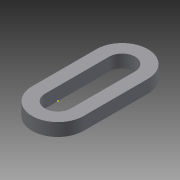
# Autodesk Inventor part: 3-2
Saved by Autodesk Inventor 2015 (Build 190159000, 159)
## iProperties
Created: 2015-09-09
Part Number: 3-2
Material: Generic
Document SubType Name: Modeling
Designer: Brandon
Density: 1 g/cm^3
Appearance: Default
Author: Brandon
Autodesk Inventor part; units mm, degrees
ref_plane "YZ Plane" through (0, 0, 0) normal (1, 0, 0) x (0, 1, 0)
ref_plane "XZ Plane" through (0, 0, 0) normal (0, 1, 0) x (-1, 0, 0)
ref_plane "XY Plane" through (0, 0, 0) normal (0, 0, 1) x (1, 0, 0)
sketch "Sketch1" plane through (0, 0, 0) normal (0, 1, 0) x (-1, 0, 0)
  circle A0 centre (0, 0) radius 25.4
  circle A1 centre (0, -63.5) radius 25.4
  line L0 (25.4, 0) -> (-25.4, 0)
  line L1 (-25.4, 0) -> (-25.4, -63.5)
  line L2 (-25.4, -63.5) -> (25.4, -63.5)
  line L3 (25.4, -63.5) -> (25.4, 0)
  dimension "d0" = 50.8
  dimension "d1" = 50.8
  dimension "d2" = 63.5
  constraints: 8 end point, 2 horizontal alignment, 2 parallel, 1 coincident, 1 horizontal, 1 perpendicular, 4 other
  measures "d2" distance of point (0, -63.5) point (0, 0)
extrude "Extrusion1" add sketch "Sketch1" along normal blind 12.7
sketch "Sketch2" plane through (0, 12.7, 0) normal (0, 1, 0) x (1, 0, 0)
  point P0 (0, 0)
sketch "Sketch3" plane through (0, 12.7, 0) normal (0, 1, 0) x (1, 0, 0)
  point P0 (0, 0)
sketch "Sketch4" plane through (0, 12.7, 0) normal (0, 1, 0) x (1, 0, 0)
  circle A0 centre (0, 0) radius 12.7
  arc A1 (-25.4, 0) -> (25.4, 0) centre (0, 0) ccw projected
  line L0 (0, 0) -> (0, 63.5)
  circle A2 centre (0, 63.5) radius 12.7
  arc A3 (25.4, 63.5) -> (-25.4, 63.5) centre (0, 63.5) ccw projected
  line L1 (-12.7, 0) -> (12.7, 0)
  line L2 (12.7, 0) -> (12.7, 63.5)
  line L3 (12.7, 63.5) -> (-12.7, 63.5)
  line L4 (-12.7, 63.5) -> (-12.7, 0)
  dimension "d5" = 12.7
  dimension "d6" = 63.5
  dimension "d7" = 12.7
  constraints: 10 end point, 2 coincident, 2 horizontal alignment, 2 parallel, 1 horizontal, 1 perpendicular, 1 vertical, 4 other
  measures "d6" distance of L0.start L0.end
extrude "Extrusion2" cut sketch "Sketch4" against normal through all
body "Solid1"
